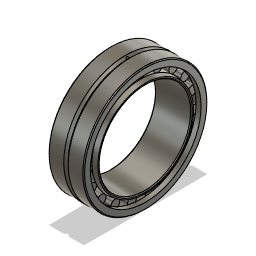
Bearing_GOST_7634-75_2_162000k (Autodesk Fusion 360 design; units mm, degrees)
Autodesk Fusion 360 part; units mm, degrees
note: some values were not read from the file. Chosen so that the rebuilt part matches the saved one: which bodies a step acts on; that a step has no effect. Set by a fixed rule: which sketch regions a step uses.
sketch "Sketch1" plane through (0, 0, 0) normal (0, 0, 1) x (1, 0, 0)
  line L0 (-85, 0) -> (85, 0)
  line L1 (-20, 50) -> (20, 51.6667)
  line L2 (20, 51.6667) -> (20, 53.9924)
  line L3 (-20, 50) -> (-20, 53.9924)
  line L4 (-14.2857, 60) -> (-14.2857, 55)
  line L5 (-14.2857, 55) -> (-2.8571, 55)
  line L6 (-2.8571, 55) -> (-2.8571, 60)
  line L7 (2.8571, 60) -> (2.8571, 55)
  line L8 (2.8571, 55) -> (14.2857, 55)
  line L9 (14.2857, 55) -> (14.2857, 60)
  line L10 (-14.2857, 65) -> (14.2857, 65)
  line L11 (20, 62.5) -> (20, 70)
  line L12 (20, 70) -> (-20, 70)
  line L13 (-20, 70) -> (-20, 62.5)
  line L14 (14.2857, 65) -> (14.2857, 60)
  line L15 (2.8571, 60) -> (2.8571, 65)
  line L16 (-2.8571, 60) -> (-2.8571, 65)
  line L17 (-14.2857, 60) -> (-14.2857, 65)
  line L18 (-8.5714, 65) -> (-8.5714, 55) construction
  line L19 (-14.2857, 60) -> (-2.8571, 60)
  line L20 (8.5714, 65) -> (8.5714, 55) construction
  line L21 (2.8571, 60) -> (14.2857, 60)
  line L22 (-5.7143, 60) -> (5.7143, 60)
  line L23 (5.7143, 60) -> (5.7143, 57.5)
  line L24 (5.7143, 57.5) -> (-5.7143, 57.5)
  line L25 (-5.7143, 57.5) -> (-5.7143, 60)
  line L26 (-2.8571, 62.5) -> (2.8571, 62.5)
  line L27 (-20, 62.5) -> (-14.2857, 62.5)
  line L28 (14.2857, 62.5) -> (20, 62.5)
  line L29 (20, 53.9924) -> (14.2857, 55)
  line L30 (-14.2857, 55) -> (-20, 53.9924)
  line L31 (-2.8571, 55) -> (2.8571, 55)
  line L32 (0, 67.5) -> (2.5, 70)
  line L33 (0, 67.5) -> (-2.5, 70)
  line L34 (0, 67.5) -> (0, 74) construction
  point P0 (0, 16.625)
  point P1 (0, 70)
  point P2 (-8.5714, 60)
  point P3 (8.5714, 60)
  point P4 (0, 60)
  point P5 (0, 65)
  point P6 (2.5, 70)
  point P7 (0, 67.5)
  dimension "d3" = 140
  dimension "d4" = 100
  dimension "d5" = 5.7143
  dimension "d6" = 11.4286
  dimension "d7" = 40
  dimension "d8" = 10
  dimension "d19" = 11.4286
  dimension "d20" = 2.5
  dimension "d22" = 103.3333
  dimension "d23" = 10
  dimension "d24" = 10
  dimension "d25" = 5
  dimension "d26" = 5
  dimension "d36" = 90
  dimension "d37" = 45
  dimension "d38" = 5
  constraint horizontal L0
  constraint midpoint L0 origin
  constraint vertical L2
  constraint vertical L3
  constraint perpendicular L4 L5
  constraint perpendicular L7 L8
  constraint horizontal L10
  constraint perpendicular L10 L11
  constraint perpendicular L11 L12
  constraint perpendicular L12 L13
  constraint vertical L2.end L11.start
  constraint vertical L3.end L13.end
  constraint midpoint L12 P1
  constraint vertical P0 P1
  constraint vertical origin P0
  constraint horizontal L4.start L6.end
  constraint horizontal L7.start L9.end
  constraint equal L5 L8
  constraint vertical L4.start L10.start
  constraint vertical L9.end L10.end
  constraint coincident L10 L15.end
  constraint perpendicular L10 L15
  constraint coincident L10 L16.end
  constraint perpendicular L10 L16
  constraint perpendicular L10 L17
  constraint coincident L10 L18.start
  constraint midpoint L5 L18.end
  constraint perpendicular L5 L18
  constraint midpoint L18 P2
  constraint coincident L17 L4.start
  constraint coincident L16 L6.end
  constraint perpendicular L16 L19
  constraint coincident P2 L19
  constraint coincident L10 L20.start
  constraint midpoint L8 L20.end
  constraint perpendicular L8 L20
  constraint coincident L15 L7.start
  constraint coincident L14 L9.end
  constraint perpendicular L14 L21
  constraint midpoint L20 P3
  constraint coincident L21 P3
  constraint horizontal L5.end L7.end
  constraint horizontal L22
  constraint vertical L23
  constraint horizontal L24
  constraint vertical L25
  constraint midpoint L22 P4
  constraint vertical P0 P4
  constraint coincident L16 L26.start
  constraint coincident L15 L26.end
  constraint perpendicular L15 L26
  constraint coincident L19 L22.start
  constraint horizontal L4.start L9.end
  constraint coincident L17 L27.end
  constraint perpendicular L17 L27
  constraint coincident L14 L28.start
  constraint perpendicular L14 L28
  constraint coincident L11.start L28.end
  constraint perpendicular L8 L9
  constraint horizontal L27.end L28.start
  constraint horizontal L26.start L27.end
  constraint midpoint L10 P5
  constraint vertical P1 P5
  constraint coincident L4.start L17.start
  constraint coincident L12 P6
  constraint vertical P1 P7
  constraint coincident P7 L32.start
  constraint coincident P6 L32
  constraint perpendicular L12 L34
  constraint coincident L12 L33.end
  measures "d5" distance of L6 L7
  measures "d6" distance of L4 L6
  measures "d7" distance of L11 L13
  measures "d8" distance of L5 L10
  measures "d19" distance of L23.end L24.end
  measures "d20" distance of L22.end L23.end
  measures "d23" angle of L5 L30
  measures "d24" angle of L8 L29
  measures "d26" vertical distance of L1.start L4.end
  measures "d36" angle of L32 L33
  measures "d37" angle of L32 L34
  measures "d38" distance of P6 L33.end
revolve "Revolve1" add sketch "Sketch1" angle 360 about axis through (-85, 0, 0) along (1, 0, 0) contours L1 L2 L3 L5 L8 L29 L30 L31 | L10 L11 L12 L13 L14 L17 L27 L28 L32 L33 | L10 L15 L16 L26 | L12 L32 L33 makes body 1 at (11.1111, -18.7406, -47.7504) makes body 2 at (-6.6667, 69.6522, -6.9697)
revolve "Revolve2" add sketch "Sketch1" angle 360 about axis through (-14.2857, 60, 0) along (1, 0, 0) separate body contours L4 L5 L6 L19 L24 L25 | L7 L8 L9 L21 L23 L24 | L6 L19 L22 L24 L25 | L7 L21 L22 L23 L24 makes body 3 at (-10.4762, 55.0062, 0.2492) makes body 4 at (6.6667, 55.0062, 0.2492)
fillet "Fillet1" radius 1 4 edges at (20, -18.6835, 48.1702) (-20, -18.0808, 46.6164) (-20, -25.3131, 65.2629) (20, -25.3131, 65.2629) on bodies 1 2
pattern_circular "C-Pattern1" count 19 over 360 about axis through (-85, 0, 0) along (1, 0, 0) of bodies 3 4 makes body 5 at (-10.4762, 43.2546, 33.9822) makes body 6 at (-10.4762, -22.324, 50.2731) makes body 7 at (-10.4762, -37.4381, 40.3006) makes body 8 at (6.6667, 51.9449, 18.0962) makes body 9 at (6.6667, 29.8769, 46.1857) makes body 10 at (6.6667, 13.2616, 53.3842) makes body 11 at (6.6667, -4.7908, 54.7978) makes body 12 at (-10.4762, -54.297, 8.8079) makes body 13 at (6.6667, -48.4951, 25.9609) makes body 14 at (-10.4762, 51.9449, 18.0962) makes body 15 at (-10.4762, 29.8769, 46.1857) makes body 16 at (-10.4762, 13.2616, 53.3842) makes body 17 at (-10.4762, -4.7908, 54.7978) makes body 18 at (-10.4762, -48.4951, 25.9609) makes body 19 at (6.6667, 43.7281, 33.4041) makes body 20 at (6.6667, -22.324, 50.2731) makes body 21 at (6.6667, -37.4381, 40.3006) makes body 22 at (6.6667, -54.297, 8.8079) makes body 23 at (-10.4762, -54.215, -9.2996) makes body 24 at (-10.4762, -48.2579, -26.3993) makes body 25 at (-10.4762, -37.0713, -40.6382) makes body 26 at (-10.4762, -21.8675, -50.4733) makes body 27 at (-10.4762, -4.294, -54.8389) makes body 28 at (-10.4762, 13.7448, -53.2619) makes body 29 at (-10.4762, 30.2942, -45.913) makes body 30 at (-10.4762, 43.5607, -33.5888) makes body 31 at (-10.4762, 52.1068, -17.6248) makes body 32 at (6.6667, -54.215, -9.2996) makes body 33 at (6.6667, -48.2579, -26.3993) makes body 34 at (6.6667, -37.0713, -40.6382) makes body 35 at (6.6667, -21.8675, -50.4733) makes body 36 at (6.6667, -4.294, -54.8389) makes body 37 at (6.6667, 13.7448, -53.2619) makes body 38 at (6.6667, 30.2942, -45.913) makes body 39 at (6.6667, 43.5607, -33.5888) makes body 40 at (6.6667, 52.1068, -17.6248)
revolve "Revolve3" add sketch "Sketch1" angle 360 about axis through (-85, 0, 0) along (1, 0, 0) separate body contours L6 L19 L22 L24 L25 | L6 L7 L22 L24 | L7 L21 L22 L23 L24 makes body 41
revolve "Revolve4" cut sketch "Sketch1" angle 360 about axis through (-85, 0, 0) along (1, 0, 0) contours L12 L32 L33 bodies 2
ref_plane "WorkPlane1" through (0, 70, 0) normal (0, 1, 0) x (0, 0, 1)
sketch "Sketch3" plane through (0, 70, 0) normal (0, 1, 0) x (1, 0, 0)
hole "Hole1" at (0, 70, 0) direction (0, -1, 0) diameter 3.2 depth 70 tip angle 180 bodies 2
pattern_circular "C-Pattern2" [no effect]
